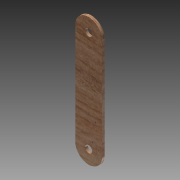
# Autodesk Inventor part: onderbeen
Saved by Autodesk Inventor 2015 (Build 190159000, 159)
## iProperties
Created: 2015-12-21
Part Number: onderbeen
Material: Generic
Document SubType Name: Modeling
Designer: david
Density: 1 g/cm^3
Appearance: Birch - Natural Polished
Author: david
Autodesk Inventor part; units mm, degrees
ref_plane "YZ Plane" through (0, 0, 0) normal (1, 0, 0) x (0, 1, 0)
ref_plane "XZ Plane" through (0, 0, 0) normal (0, 1, 0) x (-1, 0, 0)
ref_plane "XY Plane" through (0, 0, 0) normal (0, 0, 1) x (1, 0, 0)
sketch "Sketch1" plane through (0, 0, 0) normal (0, 1, 0) x (-1, 0, 0)
  line L0 (0, 0) -> (0, -120) construction
  line L1 (-20, 0) -> (-20, -120)
  line L2 (20, -120) -> (20, 0)
  arc A0 (20, 0) -> (-20, 0) centre (0, 0) ccw
  arc A1 (-20, -120) -> (20, -120) centre (0, -120) ccw
  point P0 (0, -60)
  dimension "d0" = 120
  dimension "d1" = 40
  constraints: 8 end point, 4 point on circle, 4 tangent, 2 centre point, 1 midpoint, 1 parallel, 1 vertical
  measures "d0" distance of L0.start L0.end
  measures "d1" diameter of A1
extrude "Extrusion1" add sketch "Sketch1" along normal blind 4
sketch "Sketch2" plane through (0, 4, 0) normal (0, 1, 0) x (1, 0, 0)
  circle A0 centre (0, 0) radius 5.15
  arc A1 (20, 120) -> (-20, 120) centre (0, 120) ccw projected
  circle A2 centre (0, 120) radius 5.15
  dimension "d4" = 10.3
  dimension "d5" = 10.3
  constraints: 2 centre point, 2 coincident
  measures "d4" diameter of A0
  measures "d5" diameter of A2
extrude "Extrusion2" cut sketch "Sketch2" against normal blind 4
body "Solid1"
